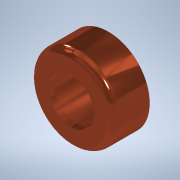
# Autodesk Inventor part: CapsuleBody
Saved by Autodesk Inventor 2020 (Build 240168000, 168)
## iProperties
Created: 2020-06-09
Part Number: CapsuleBody
Material: Copper, Wrought
Document SubType Name: Modeling
Designer: vmiguel
Density: 8.94 g/cm^3
Appearance: Copper - Polished
Author: vmiguel
Autodesk Inventor part; units mm, degrees
ref_plane "YZ Plane" through (0, 0, 0) normal (1, 0, 0) x (0, 1, 0)
ref_plane "XZ Plane" through (0, 0, 0) normal (0, 1, 0) x (-1, 0, 0)
ref_plane "XY Plane" through (0, 0, 0) normal (0, 0, 1) x (1, 0, 0)
sketch "Sketch1" plane through (0, 0, 0) normal (0, 1, 0) x (-1, 0, 0)
  line L0 (0, 0) -> (0, 10)
  line L1 (6, 10) -> (9, 10)
  line L2 (11, 8) -> (11, 0.2)
  line L3 (10.8, 0) -> (8.125, 0)
  line L4 (8.125, 0) -> (8.125, 8)
  line L5 (7.625, 8.5) -> (6, 8.5)
  line L6 (6, 8.5) -> (6, 10)
  arc A0 (11, 8) -> (9, 10) centre (9, 8) ccw
  line L7 (11, 0.2) -> (10.8, 0)
  arc A1 (8.125, 8) -> (7.625, 8.5) centre (7.625, 8) ccw
  point P0 (11, 0)
  point P1 (8.125, 8.5)
  dimension "d0" = 10
  dimension "d1" = 12
  dimension "d2" = 16.25
  dimension "d3" = 1.5
  dimension "d4" = 22
  dimension "d5" = 2
  dimension "d6" = 0.2
  dimension "d7" = 0.2
  dimension "d48" = 0.5
  constraints: 16 end point, 5 perpendicular, 4 point on circle, 4 point on line, 4 tangent, 2 centre point, 2 horizontal alignment, 1 horizontal, 1 vertical
  measures "d0" distance of L0.start L0.end
  measures "d1" diameter of L6 L0
  measures "d2" diameter of L4 L0
  measures "d3" distance of L5.end L1.start
  measures "d4" diameter of L2 L0
  measures "d5" radius of A0
  measures "d6" distance of L2.end point (11, 0)
  measures "d7" distance of L3.start point (11, 0)
  measures "d48" radius of A1
revolve "Revolution1" add sketch "Sketch1" angle 360 about axis through (0, 0, 0) along (0, 0, 1)
equation "\"d7\" = d6"
body "Solid1"
